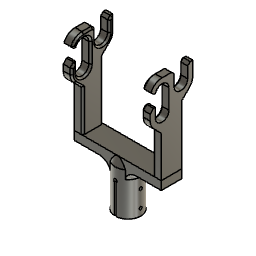
Fourche Cool Roof (Autodesk Fusion 360 design; units mm, degrees)
Autodesk Fusion 360 part; units mm, degrees
sketch "Esquisse1" plane through (0, 0, 0) normal (1, 0, 0) x (0, 1, 0)
  line L0 (25, 23) -> (27.07706, 23)
  line L1 (25, 23) -> (21, 19)
  line L2 (21, 19) -> (21, 12)
  line L3 (27.07706, 13.107708) -> (27.07706, 23)
  arc A0 (35.000001, 49.000001) -> (21.944615, 40.055386) centre (35.000001, 35.000001) ccw
  line L4 (49.000001, 35.000001) -> (49.000001, 33)
  line L5 (43.000001, 35.000001) -> (43.000001, 12)
  arc A1 (43.000001, 35.000001) -> (27.254034, 37.000001) centre (35.000001, 35.000001) ccw
  arc A2 (27.07706, 13.107708) -> (43.000001, 12) centre (35.000001, 12) ccw
  line L6 (27.254034, 37.000001) -> (25, 37.000001)
  line L7 (25, 37.000001) -> (21.944615, 40.055386)
  arc A3 (21, 12) -> (25.100505, 2.100505) centre (35.000001, 12) ccw
  line L8 (49.000001, 33) -> (49.000001, 46.032109)
  line L9 (43.002618, 49.000001) -> (46.00131, 49.000001)
  line L10 (49.000001, 46.032109) -> (46.00131, 49.000001)
  line L11 (68.000001, 49.000001) -> (70.999994, 49.000001)
  line L12 (70.999994, 32.985897) -> (70.999994, 49.000001)
  line L13 (65.000001, 46.000001) -> (68.000001, 49.000001)
  line L14 (65.000001, 33) -> (65.000001, 46.000001)
  arc A4 (49.000001, 33) -> (65.000001, 33.000001) centre (57.000001, 33.000001) ccw
  line L15 (58.000001, -55.000001) -> (34.000001, -55.000001)
  line L16 (34.000001, -55.000001) -> (34.000001, -6.79899)
  line L17 (58.000001, -55.000001) -> (58.000001, 14.201011)
  line L18 (66.899496, 23.100505) -> (58.000001, 14.201011)
  line L19 (25.100505, 2.100505) -> (34.000001, -6.79899)
  arc A5 (43.002618, 33.270688) -> (43.000001, 33.000001) centre (57.000001, 33.000001) ccw
  arc A6 (66.899496, 23.100505) -> (70.999994, 33.014104) centre (57.000001, 33.000001) ccw
  line L20 (35.000001, 49.000001) -> (43.002618, 49.000001)
  constraint concentric A0 A1
  constraint perpendicular L0 L2
  constraint concentric A2 A3
  constraint tangent L2 A3
  constraint perpendicular L0 L3
  constraint tangent L4 A3
  constraint vertical L4
  constraint tangent L5 A2
  constraint vertical L5
  constraint concentric A4 A5
  constraint tangent L8 A4
  constraint horizontal L9
  constraint tangent L14 A4
  constraint horizontal L11
  constraint perpendicular L11 L12
  constraint perpendicular L15 L16
  constraint perpendicular L15 L17
  constraint tangent L18 A5
  constraint tangent A3 L19
  constraint concentric A5 A6
  constraint tangent A0 L20
extrude "Extrusion1" add sketch "Esquisse1" along normal blind 10 contours L0 L1 L2 L3 A0 L4 L5 A1 A2 L6 L7 A3 L8 L9 L10 L11 L12 L13 L14 A4 L15 L16 L17 L18 L19 A6 L20 picked at (50.000001, -15.865993) makes body 1
chamfer "Chanfrein10" distance 2 angle 45 23 edges at (10, 23.472308, 38.527693) (10, 27.087207, 46.54936) (10, 40.500655, 49.000001) (10, 47.500655, 47.516055) (10, 36.008035, 42.936238) (10, 43.000001, 23.5) (10, 34.444808, 4.019288) (10, 49.000001, 39.516055) (10, 65.000001, 39.500001) (10, 57.000001, 25) (10, 66.500001, 47.500001) (10, 69.499998, 49.000001) (10, 70.999994, 41.007052) (10, 62.449748, 18.650758) (10, 69.937011, 27.648948) (10, 58.000001, -20.399495) (10, 34.000001, -30.899495) (10, 29.550253, -2.349242) (10, 21, 15.5) (10, 22.065687, 6.642432) (10, 23, 21) (10, 27.07706, 18.053854) (10, 26.03853, 23) on bodies 1
cylinder "CylindrePrimitive1" add diameter 3 height 30 placed x (1, 0, 0) y (0, 1, 0) z (0, 0, 1) at (0, -25, 0) separate body makes body 2
move_body "Aligner4" bodies 2 to x (1, 0, 0) y (0, 1, 0) z (0, 0, 1) at (5, 71.000001, -55.000001)
move_body "Déplacer16" bodies 2 to x (1, 0, 0) y (0, 1, 0) z (0, 0, 1) at (-1, 4.5, 0)
copy_body "CopyPasteBodies7" bodies 2 makes body 3
move_body "Déplacer17" bodies 3 to x (1, 0, 0) y (0, 1, 0) z (0, 0, 1) at (0, -9, 0)
combine "Combiner8" operation cut target body 1 tool bodies 3 2
box "BoitePrimitive1" add length 10 width 102 height 24 placed x (0, 0, -1) y (-1, 0, 0) z (0, 1, 0) at (10, 0, -35.000001) separate body makes body 4
move_body "Déplacer3" bodies 4 to x (1, 0, 0) y (0, 1, 0) z (0, 0, 1) at (0, -12, 0)
cylinder "CylindrePrimitive2" add diameter 30 height 50 placed x (1, 0, 0) y (0, 1, 0) z (0, 0, 1) at (0, 0, 0) separate body makes body 5
cylinder "CylindrePrimitive3" cut diameter 24 height 60 placed x (1, 0, 0) y (0, 1, 0) z (0, 0, 1) at (0, 0, 0) bodies 5
move_body "Aligner1" bodies 5 to x (1, 0, 0) y (0, 1, 0) z (0, 0, 1) at (-41, 0, -35.000001)
combine "Combiner2" operation add target body 4 tool bodies 5
fillet "Congé1" radius 10 2 edges at (-56, 0, -35.000001) (-26, 0, -35.000001) on bodies 4
cylinder "CylindrePrimitive4" add diameter 30 height 10 placed x (1, 0, 0) y (0, 1, 0) z (0, 0, 1) at (-41.000001, 0, 0) separate body makes body 6
move_body "Déplacer4" bodies 6 to x (1, 0, 0) y (0, 1, 0) z (0, 0, 1) at (0, 0, -45)
chamfer "Chanfrein5" distance 3 distance2 10 1 edges at (-54.984911, 5.424231, -45) measured on face at (-37.168451, 5.619851, -45) on bodies 6
combine "Combiner3" operation add target body 4 tool bodies 6
box "BoitePrimitive2" add length 36.000001 width 2 height 50 placed x (0, 0, 1) y (1, 0, 0) z (0, 1, 0) at (-42.000001, 0, 16) separate body makes body 7
cylinder "CylindrePrimitive5" add diameter 4 height 50 placed x (1, 0, 0) y (0, 0, -1) z (0, 1, 0) at (-41.000001, 0, 16) separate body makes body 8
combine "Combiner4" operation add target body 8 tool bodies 7
move_body "Déplacer5" bodies 8 to x (1, 0, 0) y (0, 1, 0) z (0, 0, 1) at (0, -24, -37)
cylinder "CylindrePrimitive6" add diameter 3.5 height 50 placed x (0, 0, -1) y (0, 1, 0) z (1, 0, 0) at (0, 0, 0) separate body makes body 9
move_body "Déplacer6" bodies 9 to x (1, 0, 0) y (0, 1, 0) z (0, 0, 1) at (-65, 0, 7)
copy_body "CopyPasteBodies2" bodies 9 makes body 10
move_body "Déplacer7" bodies 10 to x (1, 0, 0) y (0, 1, 0) z (0, 0, 1) at (0, 0, -20)
combine "Combiner5" operation cut target body 4 tool bodies 10 9 8
move_body "Déplacer8" bodies 4 to x (1, 0, 0) y (0, -1, 0) z (0, 0, -1) at (0, 0, -80.000001)
move_body "Déplacer9" bodies 1 to x (1, 0, 0) y (0, 1, 0) z (0, 0, 1) at (-92, 0, 0)
mirror "Symétrie miroir1" about plane through (-82, 0, 0) normal (1, 0, 0) of bodies 1 makes body 11
move_body "Déplacer10" bodies 11 to x (1, 0, 0) y (0, 1, 0) z (0, 0, 1) at (82, 0, 0)
cylinder "CylindrePrimitive7" add diameter 3.5 height 20 placed x (1, 0, 0) y (0, 1, 0) z (0, 0, 1) at (-75.000001, 15, 0) separate body makes body 12
move_body "Aligner5" bodies 4 to x (1, 0, 0) y (0, 1, 0) z (0, 0, 1) at (0, 46.000001, -20)
move_body "Aligner6" bodies 12 to x (1, 0, 0) y (0, 1, 0) z (0, 0, 1) at (-12.999999, 35.5, -75.000001)
copy_body "CopyPasteBodies8" bodies 12 makes body 13
move_body "Déplacer19" bodies 13 to x (1, 0, 0) y (0, 1, 0) z (0, 0, 1) at (0, -9, 0)
copy_body "CopyPasteBodies9" bodies 13 12 makes body 14 makes body 15
move_body "Déplacer20" bodies 14 15 to x (1, 0, 0) y (0, 1, 0) z (0, 0, 1) at (94, 0, 0)
combine "Combiner9" operation cut target body 4 tool bodies 13 12 15 14
